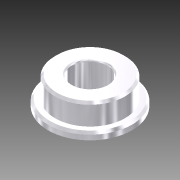
# Autodesk Inventor part: cojinete polea x
Saved by Autodesk Inventor 2012 SP2 (Build 160219200, 219)
## iProperties
Created: 2014-07-04
Part Number: cojinete polea x
Material: Default
Document SubType Name: Modeling
Designer: Principal
Density: 1 g/cm^3
Author: Principal
Autodesk Inventor part; units mm, degrees
ref_plane "YZ Plane" through (0, 0, 0) normal (1, 0, 0) x (0, 1, 0)
ref_plane "XZ Plane" through (0, 0, 0) normal (0, 1, 0) x (-1, 0, 0)
ref_plane "XY Plane" through (0, 0, 0) normal (0, 0, 1) x (1, 0, 0)
sketch "Boceto1" plane through (0, 0, 0) normal (0, 0, 1) x (1, 0, 0)
  circle A0 centre (0, 0) radius 6
  circle A1 centre (0, 0) radius 2.5
  constraints: 2 centre point, 2 coincident
extrude "Extrusión1" add sketch "Boceto1" along normal blind 4
sketch "Boceto2" plane through (0, 0, 4) normal (0, 0, 1) x (1, 0, 0)
  circle A0 centre (0, 0) radius 6 projected
  circle A1 centre (0, 0) radius 5
  constraints: 1 centre point, 1 coincident
fillet "Empalme1" radius 0.3 2 edges at (-2.5, 0, 4) (-2.5, 0, 0)
extrude "Extrusión3" cut sketch "Boceto2" against normal blind 3
chamfer "Chaflán2" distance 0.3 angle 45 2 edges at (-5, 0, 4) (-6, 0, 1)
